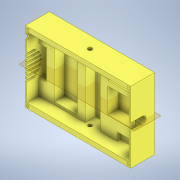
# Autodesk Inventor part: caseLowerPortion
Saved by Autodesk Inventor 2022.1 (Build 261234020, 234B)
## iProperties
Created: 2021-08-20
Part Number: caseLowerPortion
Material: PC/ABS Plastic
Document SubType Name: Modeling
Designer: robst
Density: 0.357273 g/cm^3
Appearance: Smooth - Yellow
Author: robst
Autodesk Inventor part; units mm, degrees
ref_plane "YZ Plane" through (0, 0, 0) normal (1, 0, 0) x (0, 1, 0)
ref_plane "XY Plane" through (0, 0, 0) normal (0, 0, 1) x (1, 0, 0)
sketch "Sketch1" plane through (0, 0, 0) normal (0, 0, 1) x (1, 0, 0)
  line L0 (-110.35, -74.5) -> (110.35, -74.5)
  line L1 (110.35, -74.5) -> (110.35, 74.5)
  line L2 (110.35, 74.5) -> (-110.35, 74.5)
  line L3 (-110.35, 74.5) -> (-110.35, -74.5)
  line L4 (-110.35, -74.5) -> (110.35, 74.5) construction
  line L5 (110.35, -74.5) -> (-110.35, 74.5) construction
  point P0 (0, 0)
  dimension "d0" = 220.7
  dimension "d1" = 149
  constraints: 12 end point, 2 midpoint, 2 parallel, 1 horizontal, 1 perpendicular
  measures "d0" distance of L0.start L0.end
  measures "d1" distance of L1.end L0.end
extrude "MainInnerBodyExtrusion" add sketch "Sketch1" against normal blind 50
sketch "Sketch3" plane through (0, 0, 0) normal (0, 0, 1) x (1, 0, 0)
  line L0 (37.65, -26) -> (94.65, -26)
  line L1 (94.65, -26) -> (94.65, 26)
  line L2 (94.65, 26) -> (37.65, 26)
  line L3 (37.65, 26) -> (37.65, -26)
  line L4 (37.65, -26) -> (94.65, 26) construction
  line L5 (94.65, -26) -> (37.65, 26) construction
  line L6 (110.35, -74.5) -> (110.35, 74.5) projected
  line L7 (0, 0) -> (110.35, 0) construction
  line L8 (-110.35, -74.5) -> (-110.35, 74.5) construction
  line L9 (-110.35, 74.5) -> (-110.35, -74.5) projected
  point P0 (66.15, 0)
  point P1 (66.15, 0)
  dimension "d5" = 15.7
  dimension "d6" = 52
  dimension "d7" = 57
  constraints: 14 end point, 4 midpoint, 2 parallel, 1 horizontal, 1 perpendicular, 1 point on line
  measures "d5" distance between parallel lines of L1 L6
  measures "d6" distance of L0.end L1.end
  measures "d7" distance of L1.end L2.end
extrude "HoleForCamerabase" cut sketch "Sketch3" against normal blind 47
sketch "Sketch4" plane through (0, 0, 0) normal (0, 0, 1) x (1, 0, 0)
  line L0 (0, 0) -> (-110.35, 0) construction
  line L1 (-110.35, -74.5) -> (-110.35, 74.5) construction
  line L2 (-107.35, -31) -> (-91.35, -31)
  line L3 (-91.35, -31) -> (-91.35, 31)
  line L4 (-91.35, 31) -> (-107.35, 31)
  line L5 (-107.35, 31) -> (-107.35, -31)
  line L6 (-107.35, -31) -> (-91.35, 31) construction
  line L7 (-91.35, -31) -> (-107.35, 31) construction
  point P0 (-99.35, 0)
  dimension "d13" = 16
  dimension "d14" = 62
  dimension "d15" = 3
  constraints: 14 end point, 3 midpoint, 2 parallel, 1 perpendicular, 1 point on line
  measures "d13" distance of L2.start L2.end
  measures "d14" distance of L3.end L2.end
  measures "d15" distance between parallel lines of L1 L5
extrude "HoleForFan" cut sketch "Sketch4" against normal blind 47
sketch "Sketch6" plane through (0, 0, 0) normal (0, 0, 1) x (1, 0, 0)
  line L0 (-110.35, -74.5) -> (-110.35, 74.5) construction
  line L1 (-110.35, 0) -> (110.35, 0) construction
  line L2 (110.35, 74.5) -> (110.35, -74.5) construction
  line L3 (-10.35, -64.5) -> (21.65, -64.5)
  line L4 (21.65, -64.5) -> (21.65, 64.5)
  line L5 (21.65, 64.5) -> (-10.35, 64.5)
  line L6 (-10.35, 64.5) -> (-10.35, -64.5)
  line L7 (-10.35, -64.5) -> (21.65, 64.5) construction
  line L8 (21.65, -64.5) -> (-10.35, 64.5) construction
  line L9 (37.65, -26) -> (37.65, 26) projected
  point P0 (0, 0)
  point P1 (5.65, 0)
  dimension "d20" = 32
  dimension "d21" = 129
  dimension "d88" = 16
  constraints: 14 end point, 4 midpoint, 3 parallel, 1 perpendicular, 1 point on line
  measures "d20" distance of L3.start L3.end
  measures "d21" distance of L4.end L3.end
  measures "d88" distance between parallel lines of L4 L9
extrude "HoleForPi" cut sketch "Sketch6" against normal blind 47
sketch "Sketch7" plane through (0, 0, 0) normal (0, 0, 1) x (1, 0, 0)
  line L0 (0, 0) -> (-110.35, 0) construction
  line L1 (-110.35, 74.5) -> (-110.35, -74.5) construction
  line L2 (-75.35, -59) -> (-26.35, -59)
  line L3 (-26.35, -59) -> (-26.35, 59)
  line L4 (-26.35, 59) -> (-75.35, 59)
  line L5 (-75.35, 59) -> (-75.35, -59)
  line L6 (-75.35, -59) -> (-26.35, 59) construction
  line L7 (-26.35, -59) -> (-75.35, 59) construction
  line L8 (-10.35, -64.5) -> (-10.35, 64.5) projected
  line L9 (-91.35, 31) -> (-91.35, -31) construction
  point P0 (-50.85, 0)
  dimension "d25" = 16
  dimension "d26" = 49
  dimension "d27" = 118
  constraints: 14 end point, 3 midpoint, 2 parallel, 1 perpendicular, 1 point on line
  measures "d25" distance between parallel lines of L3 L8
  measures "d26" distance of L2.start L2.end
  measures "d27" distance of L4.end L2.start
extrude "HoleForPoeAdapter" cut sketch "Sketch7" against normal blind 47
sketch "Sketch10" plane through (0, 0, 0) normal (0, 0, 1) x (1, 0, 0)
  line L0 (38.35, 36.5) -> (107.35, 36.5)
  line L1 (107.35, 36.5) -> (107.35, 64.5)
  line L2 (107.35, 64.5) -> (38.35, 64.5)
  line L3 (38.35, 64.5) -> (38.35, 36.5)
  line L4 (38.35, 36.5) -> (107.35, 64.5) construction
  line L5 (107.35, 36.5) -> (38.35, 64.5) construction
  line L6 (110.35, 74.5) -> (-110.35, 74.5) projected
  line L7 (110.35, -74.5) -> (110.35, 74.5) projected
  point P0 (0, 0)
  point P1 (72.85, 50.5)
  point P2 (94.85, 8.5)
  point P3 (107.35, 50.5)
  dimension "d36" = 69
  dimension "d37" = 28
  dimension "d85" = 3
  constraints: 12 end point, 3 midpoint, 2 parallel, 1 horizontal, 1 perpendicular, 1 other
  measures "d36" distance of L1.end L2.end
  measures "d37" distance of L0.end L1.end
extrude "HoleForThermister" cut sketch "Sketch10" against normal blind 47
sketch "Sketch11" plane through (0, 0, 0) normal (0, 0, 1) x (1, 0, 0)
  line L0 (57.35, -64.5) -> (107.35, -64.5)
  line L1 (107.35, -64.5) -> (107.35, -47.5)
  line L2 (107.35, -47.5) -> (57.35, -47.5)
  line L3 (57.35, -47.5) -> (57.35, -64.5)
  line L4 (57.35, -64.5) -> (107.35, -47.5) construction
  line L5 (107.35, -64.5) -> (57.35, -47.5) construction
  line L6 (110.35, -74.5) -> (110.35, 74.5) projected
  line L7 (-110.35, -74.5) -> (110.35, -74.5) projected
  line L8 (94.65, -26) -> (37.65, -26) projected
  line L9 (21.65, 64.5) -> (21.65, -64.5) projected
  point P0 (0, 0)
  point P1 (82.35, -56)
  point P2 (94.85, -8.5)
  point P3 (82.35, -47.5)
  point P4 (57.35, -56)
  point P5 (110.35, 74.5)
  dimension "d42" = 50
  dimension "d43" = 17
  dimension "d86" = 3
  dimension "d87" = 10
  constraints: 12 end point, 4 midpoint, 2 parallel, 1 horizontal, 1 perpendicular, 1 other
  measures "d42" distance of L0.start L0.end
  measures "d43" distance of L0.end L1.end
  measures "d87" distance between parallel lines of L7 L0
extrude "HoleForSensor" cut sketch "Sketch11" against normal blind 31.5
sketch "Sketch15" plane through (-110.35, -74.5, 0) normal (-1, 0, 0) x (0, 0, 1)
  line L0 (0, 149) -> (0, 0) projected
  line L1 (0, 149) -> (-50, 149) projected
  line L2 (-50, 0) -> (-50, 149) projected
  line L3 (0, 0) -> (-50, 0) projected
  line L4 (0, 0) -> (0, 149) projected
  line L5 (0, 100.5) -> (0, 48.5) projected
  line L6 (0, 74.5) -> (-30, 74.5) construction
  line L7 (0, 76.5) -> (-29.9333, 76.5)
  line L8 (0, 84.5) -> (-28.2843, 84.5)
  line L9 (0, 80.5) -> (-29.3939, 80.5)
  line L10 (0, 76.5) -> (0, 74.5)
  line L11 (0, 88.5) -> (-26.533, 88.5)
  line L12 (0, 92.5) -> (-24, 92.5)
  line L13 (-20.3961, 96.5) -> (0, 96.5)
  line L14 (-14.9666, 100.5) -> (0, 100.5)
  line L15 (0, 84.5) -> (0, 80.5)
  line L16 (0, 100.5) -> (0, 96.5)
  line L17 (0, 92.5) -> (0, 88.5)
  line L18 (0, 72.5) -> (-29.9333, 72.5)
  line L19 (0, 64.5) -> (-28.2843, 64.5)
  line L20 (0, 68.5) -> (-29.3939, 68.5)
  line L21 (0, 72.5) -> (0, 74.5)
  line L22 (0, 60.5) -> (-26.533, 60.5)
  line L23 (0, 56.5) -> (-24, 56.5)
  line L24 (-20.3961, 52.5) -> (0, 52.5)
  line L25 (-14.9666, 48.5) -> (0, 48.5)
  line L26 (0, 64.5) -> (0, 68.5)
  line L27 (0, 56.5) -> (0, 60.5)
  line L28 (0, 48.5) -> (0, 52.5)
  line L29 (0, 72.5) -> (0, 76.5)
  line L30 (0, 80.5) -> (0, 84.5)
  line L31 (0, 88.5) -> (0, 92.5)
  line L32 (0, 96.5) -> (0, 149)
  arc A0 (-28.2843, 84.5) -> (-29.3939, 80.5) centre (0, 74.5) ccw
  arc A1 (-14.9666, 100.5) -> (-20.3961, 96.5) centre (0, 74.5) ccw
  arc A2 (-24, 92.5) -> (-26.533, 88.5) centre (0, 74.5) ccw
  arc A3 (-29.9333, 76.5) -> (-29.9333, 72.5) centre (0, 74.5) ccw
  arc A4 (-29.3939, 68.5) -> (-28.2843, 64.5) centre (0, 74.5) ccw
  arc A5 (-26.533, 60.5) -> (-24, 56.5) centre (0, 74.5) ccw
  arc A6 (-20.3961, 52.5) -> (-14.9666, 48.5) centre (0, 74.5) ccw
  point P0 (0, 74.5)
  point P1 (0, 82)
  point P2 (0, 67.0167)
  point P3 (0, 4.25)
  point P4 (-10.198, 96.5)
  point P5 (0, 48.5)
  point P6 (0, 52.5)
  point P7 (0, 56.5)
  point P8 (0, 60.5)
  point P9 (0, 64.5)
  point P10 (0, 68.5)
  point P11 (0, 72.5)
  point P12 (0, 80.5)
  point P13 (0, 84.5)
  point P14 (0, 88.5)
  point P15 (0, 92.5)
  point P16 (0, 96.5)
  dimension "d69" = 2
  dimension "d71" = 4
  dimension "d72" = 4
  dimension "d73" = 4
  dimension "d75" = 4
  dimension "d142" = 30
  constraints: 54 end point, 15 point on circle, 15 symmetric about line, 7 centre point, 3 parallel, 3 perpendicular, 2 horizontal, 1 coincident, 1 midpoint, 1 other
  measures "d69" distance between parallel lines of L7 L6
  measures "d71" distance between parallel lines of L8 L9
  measures "d72" distance between parallel lines of L11 L8
  measures "d73" distance between parallel lines of L12 L11
  measures "d75" distance between parallel lines of L13 L14
  measures "d142" radius of A2
extrude "SlotsForRearFan" cut sketch "Sketch15" against normal up to surface (3 mm away) contours L0 L13 A1 L14 | L0 L11 A2 L12 | L25 A6 L24 L0 | L0 L9 A0 L8 | L23 A5 L22 L0 | L0 L18 A3 L7 | L19 A4 L20 L0
sketch "Sketch16" plane through (0, 0, -47) normal (0, 0, 1) x (1, 0, 0)
  line L0 (94.65, 26) -> (94.65, -26) projected
  line L1 (79.15, 10.765) -> (79.15, -11.235) construction
  line L2 (77.65, 10.765) -> (77.65, -11.235)
  line L3 (74.65, -11.235) -> (74.65, 10.765)
  line L4 (71.65, 8.7746) -> (71.65, -9.2446)
  line L5 (68.65, 3.5785) -> (68.65, -4.0485)
  line L6 (80.65, 10.765) -> (80.65, -11.235)
  line L7 (83.65, -11.235) -> (83.65, 10.765)
  line L8 (86.65, 8.7746) -> (86.65, -9.2446)
  line L9 (89.65, 3.5785) -> (89.65, -4.0485)
  line L10 (72.7991, 10.765) -> (74.65, 10.765)
  line L11 (74.65, -11.235) -> (72.7991, -11.235)
  line L12 (72.7991, -11.235) -> (71.65, -9.2446)
  line L13 (68.65, -4.0485) -> (66.4483, -0.235)
  line L14 (66.4483, -0.235) -> (68.65, 3.5785)
  line L15 (71.65, 8.7746) -> (72.7991, 10.765)
  line L16 (77.65, 10.765) -> (80.65, 10.765)
  line L17 (83.65, 10.765) -> (85.5009, 10.765)
  line L18 (85.5009, -11.235) -> (83.65, -11.235)
  line L19 (80.65, -11.235) -> (77.65, -11.235)
  line L20 (91.8517, -0.235) -> (89.65, -4.0485)
  line L21 (86.65, -9.2446) -> (85.5009, -11.235)
  line L22 (85.5009, 10.765) -> (86.65, 8.7746)
  line L23 (89.65, 3.5785) -> (91.8517, -0.235)
  point P0 (0, 0)
  point P1 (79.15, -0.235)
  point P2 (68.65, -0.235)
  dimension "d78" = 15.5
  dimension "d89" = 1.5
  dimension "d90" = 3
  dimension "d91" = 3
  dimension "d92" = 3
  constraints: 46 end point, 8 symmetric about line, 6 perpendicular, 3 horizontal, 3 midpoint, 2 vertical, 7 other
  measures "d78" distance from line of point (79.15, -0.235) L0
  measures "d89" distance between parallel lines of L2 L1
  measures "d90" distance between parallel lines of L3 L2
  measures "d91" distance between parallel lines of L4 L3
  measures "d92" distance from line of point (68.65, -0.235) L4
extrude "VentForCamera" cut sketch "Sketch16" against normal through all
sketch "Sketch18" plane through (110.35, -74.5, 0) normal (1, 0, 0) x (0, 0, -1)
  line L0 (0, 74.5) -> (29.6767, 74.5) construction
  arc A0 (24, 66.5) -> (24, 82.5) centre (24, 74.5) ccw
  line L1 (0, 0) -> (0, 149) projected
  line L2 (24, 82.5) -> (0, 82.5)
  line L3 (24, 66.5) -> (0, 66.5)
  line L4 (0, 82.5) -> (0, 66.5)
  point P0 (0, 74.5)
  dimension "d97" = 16
  dimension "d137" = 24
  constraints: 8 end point, 3 point on line, 2 perpendicular, 2 point on circle, 2 tangent, 1 centre point, 1 collinear, 1 horizontal, 1 midpoint
  measures "d97" diameter of A0
  measures "d137" distance of point (0, 74.5) A0.centre
extrude "HoleForLens" cut sketch "Sketch18" against normal up to surface (15.7 mm away)
sketch "Sketch23" plane through (0, 0, 0) normal (0, 0, 1) x (1, 0, 0)
  line L0 (-105.35, -69.5) -> (105.35, -69.5) construction
  line L1 (105.35, -69.5) -> (105.35, 69.5) construction
  line L2 (105.35, 69.5) -> (-105.35, 69.5) construction
  line L3 (-105.35, 69.5) -> (-105.35, -69.5) construction
  line L4 (-105.35, -69.5) -> (105.35, 69.5) construction
  line L5 (105.35, -69.5) -> (-105.35, 69.5) construction
  line L6 (110.35, -74.5) -> (110.35, -8) projected
  line L7 (110.35, 74.5) -> (-110.35, 74.5) projected
  point P0 (0, 0)
  dimension "d106" = 5
  dimension "d108" = 5
  constraints: 12 end point, 4 coincident, 2 midpoint, 2 parallel, 1 horizontal, 1 perpendicular
  measures "d106" distance between parallel lines of L1 L6
  measures "d108" distance between parallel lines of L2 L7
hole "Hole for 6-32 Insert" at (-105.35, 69.5, 0) at (105.35, 69.5, 0) at (105.35, -69.5, 0) at (-105.35, -69.5, 0) direction (0, 0, -1) diameter 4.7 depth 7.2 tip angle 118 counterbore diameter 5.54 counterbore depth 5.55
hole "Screw hole for 6-32 screw" at (-105.35, -69.5, 0) at (105.35, -69.5, 0) at (105.35, 69.5, 0) at (-105.35, 69.5, 0) direction (0, 0, -1) diameter 3.797 depth 15 tip angle 118 clearance for "Hex Machine Screw" size "#6" standard "Ansi Unified Screw Threads"
sketch "Sketch24" plane through (-110.35, -74.5, 0) normal (0, -1, 0) x (1, 0, 0)
  line L0 (0, -50) -> (220.7, -50) construction
  line L1 (220.7, 0) -> (205, 0) construction
  line L2 (0, 0) -> (0, -50) projected
  point P0 (110.35, 0)
  point P1 (110.35, -25)
  dimension "d143" = 25
  dimension "d147" = 110.35
  constraints: 2 other
  measures "d143" distance from line of point (110.35, -25) L0
  measures "d147" distance from line of point (110.35, -25) L2
hole "Side hole for 1-4 20 insert" at (0, -74.5, -25) direction (0, 1, 0) diameter 7.92 depth 10 tip angle 118 counterbore diameter 8.66 counterbore depth 7.41
mirror "Mirror for side insert" about plane through (0, 0, 0) normal (0, 1, 0) of "Side hole for 1-4 20 insert"
sketch "Sketch25" plane through (0, 0, 0) normal (0, 0, 1) x (1, 0, 0)
  line L0 (110.35, 74.5) -> (-110.35, 74.5) projected
  line L1 (-110.35, 74.5) -> (-110.35, 26) projected
  line L2 (-110.35, -74.5) -> (110.35, -74.5) projected
  line L3 (80.65, -11.235) -> (77.65, -11.235) projected
  line L4 (77.65, -11.235) -> (77.65, 10.765) projected
  line L5 (77.65, 10.765) -> (80.65, 10.765) projected
  line L6 (80.65, 10.765) -> (80.65, -11.235) projected
  line L7 (72.7991, 10.765) -> (74.65, 10.765) projected
  line L8 (74.65, 10.765) -> (74.65, -11.235) projected
  line L9 (74.65, -11.235) -> (72.7991, -11.235) projected
  line L10 (72.7991, -11.235) -> (71.65, -9.2446) projected
  line L11 (71.65, -9.2446) -> (71.65, 8.7746) projected
  line L12 (71.65, 8.7746) -> (72.7991, 10.765) projected
  line L13 (86.65, 8.7746) -> (86.65, -9.2446) projected
  line L14 (86.65, -9.2446) -> (85.5009, -11.235) projected
  line L15 (85.5009, -11.235) -> (83.65, -11.235) projected
  line L16 (83.65, -11.235) -> (83.65, 10.765) projected
  line L17 (83.65, 10.765) -> (85.5009, 10.765) projected
  line L18 (85.5009, 10.765) -> (86.65, 8.7746) projected
  line L19 (68.65, 3.5785) -> (68.65, -4.0485) projected
  line L20 (68.65, -4.0485) -> (66.4483, -0.235) projected
  line L21 (66.4483, -0.235) -> (68.65, 3.5785) projected
  line L22 (91.8517, -0.235) -> (89.65, -4.0485) projected
  line L23 (89.65, -4.0485) -> (89.65, 3.5785) projected
  line L24 (89.65, 3.5785) -> (91.8517, -0.235) projected
  line L25 (94.65, 26) -> (94.65, -26) projected
  line L26 (37.65, 26) -> (94.65, 26) projected
  line L27 (37.65, -26) -> (37.65, 26) projected
  line L28 (94.65, -26) -> (37.65, -26) projected
  line L29 (110.35, -74.5) -> (110.35, -8) projected
  line L30 (110.35, 8) -> (110.35, 74.5) projected
  line L31 (-107.35, -64.5) -> (107.35, -64.5)
  line L32 (107.35, -64.5) -> (107.35, 64.5)
  line L33 (107.35, 64.5) -> (-107.35, 64.5)
  line L34 (-107.35, 64.5) -> (-107.35, -64.5)
  line L35 (-107.35, -64.5) -> (107.35, 64.5) construction
  line L36 (107.35, -64.5) -> (-107.35, 64.5) construction
  line L37 (-26.35, 59) -> (-26.35, -59) projected
  point P0 (0, 0)
  dimension "d138" = 10
  dimension "d139" = 3
  constraints: 12 end point, 2 midpoint, 2 parallel, 2 perpendicular
  measures "d138" distance between parallel lines of L2 L31
  measures "d139" distance between parallel lines of L1 L34
extrude "Extrusion18" cut sketch "Sketch25" against normal blind 25 contours L34 L33 L32 L31
sketch "Sketch26" plane through (-110.35, -74.5, -50) normal (-1, 0, 0) x (0, 0, 1)
  arc A0 (50, 124) -> (50, 134) centre (50, 129) ccw
  circle A1 centre (50, 129) radius 5
  point P0 (50, 74.5)
  point P1 (50, 124)
  constraints: 2 centre point, 2 point on circle, 1 coincident, 1 concentric, 4 other
extrude "Extrusion19" cut sketch "Sketch26" against normal up to surface (3 mm away)
sketch "Sketch28" plane through (-110.35, -74.5, 0) normal (0, -1, 0) x (1, 0, 0)
  line L0 (220.7, -50) -> (0, -50) projected
  line L1 (100, -25) -> (3, -25) projected
  line L2 (84, -25) -> (84, -47) projected
  line L3 (100, -25) -> (100, -47) projected
  line L4 (167.7, -25) -> (132, -25) projected
  line L5 (132, -25) -> (132, -47) projected
  line L6 (217.7, -25) -> (167.7, -25) projected
  line L7 (148, -25) -> (148, -47) projected
  line L8 (84, -47) -> (35, -47) projected
  line L9 (205, -47) -> (148, -47) projected
  line L10 (132, -47) -> (100, -47) projected
  line L11 (100, -47) -> (132, -47) construction
  line L12 (84, -25) -> (100, -47) construction
  line L13 (100, -25) -> (84, -47) construction
  line L14 (148, -25) -> (148, -47) construction
  line L15 (132, -25) -> (148, -47) construction
  line L16 (148, -25) -> (132, -47) construction
  point P0 (110.35, 0)
  point P1 (92, -36)
  point P2 (140, -36)
  constraints: 8 end point, 2 midpoint
hole "Hole5" at (29.65, -74.5, -36) at (-18.35, -74.5, -36) direction (0, 1, 0) diameter 6.756 depth 74.5 tip angle 118 clearance for "Flat Head Machine Screw (82)" size "1/4" standard "Ansi Unified Screw Threads"
hole "Hole6" at (-18.35, -74.5, -36) at (29.65, -74.5, -36) direction (0, 1, 0) diameter 7.92 depth 10 tip angle 118 counterbore diameter 8.66 counterbore depth 7.41
equation "\"d0\" = newCaseLength"
equation "\"d1\" = caseWidth"
equation "\"d2\" = caseDepth"
equation "\"d5\" = lensLength"
equation "\"d6\" = cameraWidth"
equation "\"d7\" = cameraLength"
equation "\"d8\" = maxComponentDepth"
equation "\"d13\" = fanDepth"
equation "\"d14\" = fanWidth"
equation "\"d15\" = rearWallThickness"
equation "\"d16\" = maxComponentDepth"
equation "\"d20\" = piCaseDepth"
equation "\"d21\" = piCaseLength"
equation "\"d88\" = minDelta"
equation "\"d22\" = maxComponentDepth"
equation "\"d25\" = minDelta"
equation "\"d26\" = poeWidth"
equation "\"d27\" = poeLength"
equation "\"d28\" = maxComponentDepth"
equation "\"d36\" = thermisterLength"
equation "\"d37\" = thermisterWidth"
equation "\"d85\" = frontWallThickness"
equation "\"d38\" = maxComponentDepth"
equation "\"d42\" = sensorLength"
equation "\"d43\" = sensorWidth"
equation "\"d86\" = frontWallThickness"
equation "\"d87\" = outsideWallThickness"
equation "\"d46\" = cutoutDepth"
equation "\"outsideWallThickness\" = 10"
equation "\"caseWidth\" = piCaseLength + 2 * outsideWallThickness"
equation "\"oneHalfCaseDepth\" = piCaseWidth"
equation "\"caseLength\" = 189.7"
equation "\"lensLength\" = 15.7"
equation "\"piCaseWidth\" = 63"
equation "\"piCaseDepth\" = 32"
equation "\"poeDepth\" = 38"
equation "\"piEthernetCableReliefLength\" = 35"
equation "\"poeEthernetCableReliefLength\" = 35"
equation "\"thermisterDepth\" = 18"
equation "\"sensorDepth\" = 11"
equation "\"cutoutDepth\" = 0.5 * piCaseWidth"
equation "\"thickenDistance\" = 1"
equation "\"bottomOfCaseWallThickness\" = 3"
equation "\"rearWallThickness\" = 3"
equation "\"maxComponentDepth\" = extraCutoutDepth + 0.5 * piCaseWidth"
equation "\"caseDepth\" = maxComponentDepth + bottomOfCaseWallThickness"
equation "\"minDelta\" = 16"
equation "\"fanCutoutDepth\" = 0.5 * fanLength + extraCutoutDepth + thickenDistance"
equation "\"newCaseLength\" = cameraLength + piCaseDepth + fanDepth + poeWidth + rearWallThickness + 3 * minDelta + lensLength"
equation "\"frontWallThickness\" = 3"
equation "\"d95\" = lensDiameter"
equation "\"extraCutoutDepth\" = 15.5"
equation "\"cameraWidth\" = 52"
equation "\"cameraLength\" = 57"
equation "\"fanDepth\" = 16"
equation "\"fanWidth\" = 62"
equation "\"piCaseLength\" = 129"
equation "\"poeWidth\" = 49"
equation "\"poeLength\" = 118"
equation "\"thermisterLength\" = 69"
equation "\"thermisterWidth\" = 28"
equation "\"sensorLength\" = 50"
equation "\"sensorWidth\" = 17"
equation "\"fanLength\" = 60"
equation "\"lensDiameter\" = 15"
body "Solid1"
